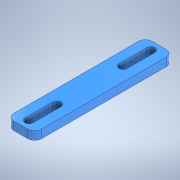
# Autodesk Inventor part: Carriage_Horizontal_Spacer
Saved by Autodesk Inventor 2021 (Build 250183000, 183)
## iProperties
Created: 2021-10-04
Part Number: Carriage_Horizontal_Spacer
Material: Generic
Document SubType Name: Modeling
Designer: Jorian Bruslind
Density: 1 g/cm^3
Appearance: Cyan
Author: Jorian Bruslind
Autodesk Inventor part; units mm, degrees
ref_plane "YZ Plane" through (0, 0, 0) normal (1, 0, 0) x (0, 1, 0)
ref_plane "XZ Plane" through (0, 0, 0) normal (0, 1, 0) x (-1, 0, 0)
ref_plane "XY Plane" through (0, 0, 0) normal (0, 0, 1) x (1, 0, 0)
sketch "Sketch1" plane through (0, 0, 0) normal (0, 1, 0) x (-1, 0, 0)
  line L0 (0, 0) -> (-20, 0)
  line L1 (-20, 0) -> (-20, -100)
  line L2 (-20, -100) -> (0, -100)
  line L3 (0, -100) -> (0, 0)
  line L4 (-10, 0) -> (-10, -6)
  line L5 (-10, -6) -> (60, -6) construction
  line L6 (-10, -6) -> (-10, -26) construction
  line L7 (-13, -6) -> (-13, -26)
  line L8 (-7, -26) -> (-7, -6)
  arc A0 (-7, -6) -> (-13, -6) centre (-10, -6) ccw
  arc A1 (-13, -26) -> (-7, -26) centre (-10, -26) ccw
  line L9 (-10, -100) -> (-10, -94)
  line L10 (-10, -94) -> (-10, -74) construction
  line L11 (-7, -94) -> (-7, -74)
  line L12 (-13, -74) -> (-13, -94)
  arc A2 (-13, -94) -> (-7, -94) centre (-10, -94) ccw
  arc A3 (-7, -74) -> (-13, -74) centre (-10, -74) ccw
  point P0 (-10, -16)
  point P1 (-10, -84)
  dimension "d0" = 20
  dimension "d1" = 100
  dimension "d2" = 6
  dimension "d9" = 20
  dimension "d10" = 6
  dimension "d11" = 6
  dimension "d12" = 20
  dimension "d13" = 6
  constraints: 30 end point, 8 point on circle, 8 tangent, 4 centre point, 4 midpoint, 4 parallel, 4 vertical, 2 horizontal, 1 perpendicular
  measures "d0" distance of L2.end L1.end
  measures "d1" distance of L1.end L0.end
  measures "d2" distance of L4.start L4.end
  measures "d9" distance of L4.end L6.end
  measures "d10" diameter of A1
  measures "d11" distance of L9.start L9.end
  measures "d12" distance of L9.end L10.end
  measures "d13" diameter of A3
extrude "Extrusion1" add sketch "Sketch1" along normal blind 6
fillet "Fillet1" radius 5 4 edges at (20, 3, 0) (0, 3, 0) (20, 3, -100) (0, 3, -100)
body "Solid1"
